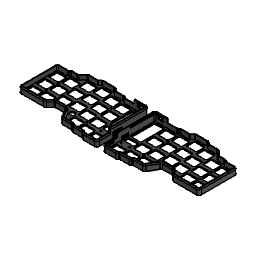
mriya-bumper-mjf-v1.09 (Autodesk Fusion 360 design; units mm, degrees)
Autodesk Fusion 360 part; units mm, degrees
(part 1 of 2)
sketch "mriya" plane through (0, 0, 0) normal (0, 0, 1) x (1, 0, 0)
  line L0 (-101.0213, 15.6719) -> (-94.7787, 21.9145) construction
  line L1 (-26.4858, 1.079) -> (-27.6142, 2.2074) construction
  line L2 (-138.1, 14.7932) -> (-103.1426, 14.7932) construction
  line L3 (-44.0716, 2.7932) -> (-29.0284, 2.7932) construction
  line L4 (-8.6, 0.4932) -> (-25.0716, 0.4932) construction
  line L5 (-64.4741, 6.1094) -> (-72.7517, 20.7608) construction
  line L6 (-45.4858, 3.379) -> (-46.6142, 4.5074) construction
  line L7 (-122.6142, 71.579) -> (-121.4858, 72.7074) construction
  line L8 (-101.0716, 81.2932) -> (-87.2284, 81.2932) construction
  line L9 (-138.1, 70.9932) -> (-124.0284, 70.9932) construction
  line L10 (-92.6574, 22.7932) -> (-76.2344, 22.7932) construction
  line L11 (-48.0284, 5.0932) -> (-62.7328, 5.0932) construction
  line L12 (-82.0716, 84.7932) -> (-64.7284, 84.7932) construction
  line L13 (-58.5716, 80.2932) -> (-45.7284, 80.2932) construction
  line L14 (-24.1, 19.4932) -> (-7.1, 19.4932) construction
  line L15 (-25.6, 20.9932) -> (-25.6, 77.9932) construction
  line L16 (-83.4858, 84.2074) -> (-85.8142, 81.879) construction
  line L17 (-63.3142, 84.2074) -> (-59.9858, 80.879) construction
  line L18 (-139.6, 69.4932) -> (-139.6, 16.2932) construction
  line L19 (-43.1858, 78.579) -> (-44.3142, 79.7074) construction
  line L20 (-99.4, 40.3932) -> (-99.4, 27.9932) construction
  line L21 (-98.6, 41.1932) -> (-86.2, 41.1932) construction
  line L22 (-98.6, 27.1932) -> (-86.2, 27.1932) construction
  line L23 (-85.4, 40.3932) -> (-85.4, 27.9932) construction
  line L24 (-42.4, 56.0932) -> (-42.4, 43.6932) construction
  line L25 (-41.6, 56.8932) -> (-29.2, 56.8932) construction
  line L26 (-41.6, 42.8932) -> (-29.2, 42.8932) construction
  line L27 (-28.4, 56.0932) -> (-28.4, 43.6932) construction
  line L28 (-61.4, 58.3932) -> (-61.4, 45.9932) construction
  line L29 (-60.6, 59.1932) -> (-48.2, 59.1932) construction
  line L30 (-60.6, 45.1932) -> (-48.2, 45.1932) construction
  line L31 (-47.4, 58.3932) -> (-47.4, 45.9932) construction
  line L32 (-137.4, 68.0932) -> (-137.4, 55.6932) construction
  line L33 (-136.6, 68.8932) -> (-124.2, 68.8932) construction
  line L34 (-136.6, 54.8932) -> (-124.2, 54.8932) construction
  line L35 (-123.4, 68.0932) -> (-123.4, 55.6932) construction
  line L36 (-61.4, 39.3932) -> (-61.4, 26.9932) construction
  line L37 (-60.6, 40.1932) -> (-48.2, 40.1932) construction
  line L38 (-60.6, 26.1932) -> (-48.2, 26.1932) construction
  line L39 (-47.4, 39.3932) -> (-47.4, 26.9932) construction
  line L40 (-42.4, 18.0932) -> (-42.4, 5.6932) construction
  line L41 (-41.6, 18.8932) -> (-29.2, 18.8932) construction
  line L42 (-41.6, 4.8932) -> (-29.2, 4.8932) construction
  line L43 (-28.4, 18.0932) -> (-28.4, 5.6932) construction
  line L44 (-23.4, 15.7932) -> (-23.4, 3.3932) construction
  line L45 (-22.6, 16.5932) -> (-10.2, 16.5932) construction
  line L46 (-22.6, 2.5932) -> (-10.2, 2.5932) construction
  line L47 (-9.4, 15.7932) -> (-9.4, 3.3932) construction
  line L48 (-137.4, 49.0932) -> (-137.4, 36.6932) construction
  line L49 (-136.6, 49.8932) -> (-124.2, 49.8932) construction
  line L50 (-136.6, 35.8932) -> (-124.2, 35.8932) construction
  line L51 (-123.4, 49.0932) -> (-123.4, 36.6932) construction
  line L52 (-118.4, 51.3932) -> (-118.4, 38.9932) construction
  line L53 (-117.6, 52.1932) -> (-105.2, 52.1932) construction
  line L54 (-117.6, 38.1932) -> (-105.2, 38.1932) construction
  line L55 (-104.4, 51.3932) -> (-104.4, 38.9932) construction
  line L56 (-137.4, 30.0932) -> (-137.4, 17.6932) construction
  line L57 (-136.6, 30.8932) -> (-124.2, 30.8932) construction
  line L58 (-136.6, 16.8932) -> (-124.2, 16.8932) construction
  line L59 (-123.4, 30.0932) -> (-123.4, 17.6932) construction
  line L60 (-61.4, 20.3932) -> (-61.4, 7.9932) construction
  line L61 (-60.6, 21.1932) -> (-48.2, 21.1932) construction
  line L62 (-60.6, 7.1932) -> (-48.2, 7.1932) construction
  line L63 (-47.4, 20.3932) -> (-47.4, 7.9932) construction
  line L64 (-80.4, 43.8932) -> (-80.4, 31.4932) construction
  line L65 (-79.6, 44.6932) -> (-67.2, 44.6932) construction
  line L66 (-79.6, 30.6932) -> (-67.2, 30.6932) construction
  line L67 (-66.4, 43.8932) -> (-66.4, 31.4932) construction
  line L68 (-80.4, 81.8932) -> (-80.4, 69.4932) construction
  line L69 (-79.6, 82.6932) -> (-67.2, 82.6932) construction
  line L70 (-79.6, 68.6932) -> (-67.2, 68.6932) construction
  line L71 (-66.4, 81.8932) -> (-66.4, 69.4932) construction
  line L72 (-42.4, 37.0932) -> (-42.4, 24.6932) construction
  line L73 (-41.6, 37.8932) -> (-29.2, 37.8932) construction
  line L74 (-41.6, 23.8932) -> (-29.2, 23.8932) construction
  line L75 (-28.4, 37.0932) -> (-28.4, 24.6932) construction
  line L76 (-118.4, 32.3932) -> (-118.4, 19.9932) construction
  line L77 (-117.6, 33.1932) -> (-105.2, 33.1932) construction
  line L78 (-117.6, 19.1932) -> (-105.2, 19.1932) construction
  line L79 (-104.4, 32.3932) -> (-104.4, 19.9932) construction
  line L80 (-61.4, 77.3932) -> (-61.4, 64.9932) construction
  line L81 (-60.6, 78.1932) -> (-48.2, 78.1932) construction
  line L82 (-60.6, 64.1932) -> (-48.2, 64.1932) construction
  line L83 (-47.4, 77.3932) -> (-47.4, 64.9932) construction
  line L84 (-42.4, 75.0932) -> (-42.4, 62.6932) construction
  line L85 (-41.6, 75.8932) -> (-29.2, 75.8932) construction
  line L86 (-41.6, 61.8932) -> (-29.2, 61.8932) construction
  line L87 (-28.4, 75.0932) -> (-28.4, 62.6932) construction
  line L88 (-118.4, 70.3932) -> (-118.4, 57.9932) construction
  line L89 (-117.6, 71.1932) -> (-105.2, 71.1932) construction
  line L90 (-117.6, 57.1932) -> (-105.2, 57.1932) construction
  line L91 (-104.4, 70.3932) -> (-104.4, 57.9932) construction
  line L92 (-99.4, 59.3932) -> (-99.4, 46.9932) construction
  line L93 (-98.6, 60.1932) -> (-86.2, 60.1932) construction
  line L94 (-98.6, 46.1932) -> (-86.2, 46.1932) construction
  line L95 (-85.4, 59.3932) -> (-85.4, 46.9932) construction
  line L96 (-80.4, 62.8932) -> (-80.4, 50.4932) construction
  line L97 (-79.6, 63.6932) -> (-67.2, 63.6932) construction
  line L98 (-79.6, 49.6932) -> (-67.2, 49.6932) construction
  line L99 (-66.4, 62.8932) -> (-66.4, 50.4932) construction
  line L100 (-99.4, 78.3932) -> (-99.4, 65.9932) construction
  line L101 (-98.6, 79.1932) -> (-86.2, 79.1932) construction
  line L102 (-98.6, 65.1932) -> (-86.2, 65.1932) construction
  line L103 (-85.4, 78.3932) -> (-85.4, 65.9932) construction
  circle A0 centre (-120.9, 53.5432) radius 1.65
  circle A1 centre (-120.9, 34.5432) radius 1.65
  circle A2 centre (-68.5, 23.5932) radius 4
  circle A3 centre (-44.9, 22.5432) radius 1.65
  circle A4 centre (-44.9, 60.5432) radius 1.65
  arc A5 (-43.1858, 78.579) -> (-41.7716, 77.9932) centre (-41.7716, 79.9932) ccw construction
  arc A6 (-44.3142, 79.7074) -> (-45.7284, 80.2932) centre (-45.7285, 78.2931) ccw construction
  arc A7 (-59.9858, 80.879) -> (-58.5716, 80.2932) centre (-58.5716, 82.2931) ccw construction
  arc A8 (-63.3142, 84.2074) -> (-64.7284, 84.7932) centre (-64.7285, 82.7931) ccw construction
  arc A9 (-82.0716, 84.7932) -> (-83.4858, 84.2074) centre (-82.0716, 82.7933) ccw construction
  arc A10 (-87.2284, 81.2932) -> (-85.8142, 81.879) centre (-87.2284, 83.2932) ccw construction
  arc A11 (-101.0716, 81.2932) -> (-102.4858, 80.7074) centre (-101.0716, 79.2933) ccw construction
  arc A12 (-120.0716, 73.2932) -> (-121.4858, 72.7074) centre (-120.0716, 71.2933) ccw construction
  arc A13 (-124.0284, 70.9932) -> (-122.6142, 71.579) centre (-124.0284, 72.9932) ccw construction
  arc A14 (-138.1, 70.9932) -> (-139.6, 69.4932) centre (-138.1, 69.4932) ccw construction
  arc A15 (-139.6, 16.2932) -> (-138.1, 14.7932) centre (-138.1, 16.2932) ccw construction
  arc A16 (-103.1426, 14.7932) -> (-101.0213, 15.6719) centre (-103.1426, 17.7931) ccw construction
  arc A17 (-92.6574, 22.7932) -> (-94.7787, 21.9145) centre (-92.6573, 19.7931) ccw construction
  arc A18 (-72.7517, 20.7608) -> (-76.2344, 22.7932) centre (-76.2344, 18.793) ccw construction
  arc A19 (-64.4741, 6.1094) -> (-62.7328, 5.0932) centre (-62.7328, 7.0932) ccw construction
  arc A20 (-46.6142, 4.5074) -> (-48.0284, 5.0932) centre (-48.0284, 3.0933) ccw construction
  arc A21 (-45.4858, 3.379) -> (-44.0716, 2.7932) centre (-44.0715, 4.7933) ccw construction
  arc A22 (-27.6142, 2.2074) -> (-29.0284, 2.7932) centre (-29.0284, 0.7933) ccw construction
  arc A23 (-26.4858, 1.079) -> (-25.0716, 0.4932) centre (-25.0715, 2.4933) ccw construction
  arc A24 (-8.6, 0.4932) -> (-7.1, 1.9932) centre (-8.6, 1.9932) ccw construction
  arc A25 (-25.6, 20.9932) -> (-24.1, 19.4932) centre (-24.1, 20.9932) ccw construction
  line L104 (-7.1, 1.9932) -> (-7.1, 76.4932) construction
  line L105 (-41.7716, 77.9932) -> (-8.6, 77.9932) construction
  arc A26 (-7.1, 76.4932) -> (-8.6, 77.9932) centre (-8.6, 76.4932) ccw construction
  arc A27 (-136.6, 68.8932) -> (-137.4, 68.0932) centre (-136.6, 68.0932) ccw construction
  arc A28 (-123.4, 68.0932) -> (-124.2, 68.8932) centre (-124.2, 68.0932) ccw construction
  arc A29 (-124.2, 54.8932) -> (-123.4, 55.6932) centre (-124.2, 55.6932) ccw construction
  arc A30 (-137.4, 55.6932) -> (-136.6, 54.8932) centre (-136.6, 55.6932) ccw construction
  arc A31 (-136.6, 49.8932) -> (-137.4, 49.0932) centre (-136.6, 49.0932) ccw construction
  arc A32 (-123.4, 49.0932) -> (-124.2, 49.8932) centre (-124.2, 49.0932) ccw construction
  arc A33 (-124.2, 35.8932) -> (-123.4, 36.6932) centre (-124.2, 36.6932) ccw construction
  arc A34 (-137.4, 36.6932) -> (-136.6, 35.8932) centre (-136.6, 36.6932) ccw construction
  arc A35 (-136.6, 30.8932) -> (-137.4, 30.0932) centre (-136.6, 30.0932) ccw construction
  arc A36 (-123.4, 30.0932) -> (-124.2, 30.8932) centre (-124.2, 30.0932) ccw construction
  arc A37 (-124.2, 16.8932) -> (-123.4, 17.6932) centre (-124.2, 17.6932) ccw construction
  arc A38 (-137.4, 17.6932) -> (-136.6, 16.8932) centre (-136.6, 17.6932) ccw construction
  arc A39 (-118.4, 19.9932) -> (-117.6, 19.1932) centre (-117.6, 19.9932) ccw construction
  arc A40 (-105.2, 19.1932) -> (-104.4, 19.9932) centre (-105.2, 19.9932) ccw construction
  arc A41 (-104.4, 32.3932) -> (-105.2, 33.1932) centre (-105.2, 32.3932) ccw construction
  arc A42 (-117.6, 33.1932) -> (-118.4, 32.3932) centre (-117.6, 32.3932) ccw construction
  arc A43 (-105.2, 38.1932) -> (-104.4, 38.9932) centre (-105.2, 38.9932) ccw construction
  arc A44 (-118.4, 38.9932) -> (-117.6, 38.1932) centre (-117.6, 38.9932) ccw construction
  arc A45 (-117.6, 52.1932) -> (-118.4, 51.3932) centre (-117.6, 51.3932) ccw construction
  arc A46 (-104.4, 51.3932) -> (-105.2, 52.1932) centre (-105.2, 51.3932) ccw construction
  arc A47 (-118.4, 57.9932) -> (-117.6, 57.1932) centre (-117.6, 57.9932) ccw construction
  arc A48 (-105.2, 57.1932) -> (-104.4, 57.9932) centre (-105.2, 57.9932) ccw construction
  arc A49 (-104.4, 70.3932) -> (-105.2, 71.1932) centre (-105.2, 70.3932) ccw construction
  arc A50 (-117.6, 71.1932) -> (-118.4, 70.3932) centre (-117.6, 70.3932) ccw construction
  arc A51 (-98.6, 79.1932) -> (-99.4, 78.3932) centre (-98.6, 78.3932) ccw construction
  arc A52 (-85.4, 78.3932) -> (-86.2, 79.1932) centre (-86.2, 78.3932) ccw construction
  arc A53 (-86.2, 65.1932) -> (-85.4, 65.9932) centre (-86.2, 65.9932) ccw construction
  arc A54 (-99.4, 65.9932) -> (-98.6, 65.1932) centre (-98.6, 65.9932) ccw construction
  arc A55 (-98.6, 60.1932) -> (-99.4, 59.3932) centre (-98.6, 59.3932) ccw construction
  arc A56 (-85.4, 59.3932) -> (-86.2, 60.1932) centre (-86.2, 59.3932) ccw construction
  arc A57 (-86.2, 46.1932) -> (-85.4, 46.9932) centre (-86.2, 46.9932) ccw construction
  arc A58 (-99.4, 46.9932) -> (-98.6, 46.1932) centre (-98.6, 46.9932) ccw construction
  arc A59 (-98.6, 41.1932) -> (-99.4, 40.3932) centre (-98.6, 40.3932) ccw construction
  arc A60 (-99.4, 27.9932) -> (-98.6, 27.1932) centre (-98.6, 27.9932) ccw construction
  arc A61 (-86.2, 27.1932) -> (-85.4, 27.9932) centre (-86.2, 27.9932) ccw construction
  arc A62 (-85.4, 40.3932) -> (-86.2, 41.1932) centre (-86.2, 40.3932) ccw construction
  arc A63 (-80.4, 31.4932) -> (-79.6, 30.6932) centre (-79.6, 31.4932) ccw construction
  arc A64 (-79.6, 44.6932) -> (-80.4, 43.8932) centre (-79.6, 43.8932) ccw construction
  arc A65 (-66.4, 43.8932) -> (-67.2, 44.6932) centre (-67.2, 43.8932) ccw construction
  arc A66 (-67.2, 30.6932) -> (-66.4, 31.4932) centre (-67.2, 31.4932) ccw construction
  arc A67 (-67.2, 49.6932) -> (-66.4, 50.4932) centre (-67.2, 50.4932) ccw construction
  arc A68 (-80.4, 50.4932) -> (-79.6, 49.6932) centre (-79.6, 50.4932) ccw construction
  arc A69 (-79.6, 63.6932) -> (-80.4, 62.8932) centre (-79.6, 62.8932) ccw construction
  arc A70 (-66.4, 62.8932) -> (-67.2, 63.6932) centre (-67.2, 62.8932) ccw construction
  arc A71 (-67.2, 68.6932) -> (-66.4, 69.4932) centre (-67.2, 69.4932) ccw construction
  arc A72 (-80.4, 69.4932) -> (-79.6, 68.6932) centre (-79.6, 69.4932) ccw construction
  arc A73 (-79.6, 82.6932) -> (-80.4, 81.8932) centre (-79.6, 81.8932) ccw construction
  arc A74 (-66.4, 81.8932) -> (-67.2, 82.6932) centre (-67.2, 81.8932) ccw construction
  arc A75 (-60.6, 78.1932) -> (-61.4, 77.3932) centre (-60.6, 77.3932) ccw construction
  arc A76 (-61.4, 64.9932) -> (-60.6, 64.1932) centre (-60.6, 64.9932) ccw construction
  arc A77 (-48.2, 64.1932) -> (-47.4, 64.9932) centre (-48.2, 64.9932) ccw construction
  arc A78 (-47.4, 77.3932) -> (-48.2, 78.1932) centre (-48.2, 77.3932) ccw construction
  arc A79 (-47.4, 58.3932) -> (-48.2, 59.1932) centre (-48.2, 58.3932) ccw construction
  arc A80 (-60.6, 59.1932) -> (-61.4, 58.3932) centre (-60.6, 58.3932) ccw construction
  arc A81 (-61.4, 45.9932) -> (-60.6, 45.1932) centre (-60.6, 45.9932) ccw construction
  arc A82 (-48.2, 45.1932) -> (-47.4, 45.9932) centre (-48.2, 45.9932) ccw construction
  arc A83 (-47.4, 39.3932) -> (-48.2, 40.1932) centre (-48.2, 39.3932) ccw construction
  arc A84 (-60.6, 40.1932) -> (-61.4, 39.3932) centre (-60.6, 39.3932) ccw construction
  arc A85 (-61.4, 26.9932) -> (-60.6, 26.1932) centre (-60.6, 26.9932) ccw construction
  arc A86 (-48.2, 26.1932) -> (-47.4, 26.9932) centre (-48.2, 26.9932) ccw construction
  arc A87 (-47.4, 20.3932) -> (-48.2, 21.1932) centre (-48.2, 20.3932) ccw construction
  arc A88 (-60.6, 21.1932) -> (-61.4, 20.3932) centre (-60.6, 20.3932) ccw construction
  arc A89 (-61.4, 7.9932) -> (-60.6, 7.1932) centre (-60.6, 7.9932) ccw construction
  arc A90 (-48.2, 7.1932) -> (-47.4, 7.9932) centre (-48.2, 7.9932) ccw construction
  arc A91 (-42.4, 5.6932) -> (-41.6, 4.8932) centre (-41.6, 5.6932) ccw construction
  arc A92 (-29.2, 4.8932) -> (-28.4, 5.6932) centre (-29.2, 5.6932) ccw construction
  arc A93 (-28.4, 18.0932) -> (-29.2, 18.8932) centre (-29.2, 18.0932) ccw construction
  arc A94 (-41.6, 18.8932) -> (-42.4, 18.0932) centre (-41.6, 18.0932) ccw construction
  arc A95 (-23.4, 3.3932) -> (-22.6, 2.5932) centre (-22.6, 3.3932) ccw construction
  arc A96 (-10.2, 2.5932) -> (-9.4, 3.3932) centre (-10.2, 3.3932) ccw construction
  arc A97 (-9.4, 15.7932) -> (-10.2, 16.5932) centre (-10.2, 15.7932) ccw construction
  arc A98 (-22.6, 16.5932) -> (-23.4, 15.7932) centre (-22.6, 15.7932) ccw construction
  arc A99 (-29.2, 23.8932) -> (-28.4, 24.6932) centre (-29.2, 24.6932) ccw construction
  arc A100 (-42.4, 24.6932) -> (-41.6, 23.8932) centre (-41.6, 24.6932) ccw construction
  arc A101 (-41.6, 37.8932) -> (-42.4, 37.0932) centre (-41.6, 37.0932) ccw construction
  arc A102 (-28.4, 37.0932) -> (-29.2, 37.8932) centre (-29.2, 37.0932) ccw construction
  arc A103 (-29.2, 42.8932) -> (-28.4, 43.6932) centre (-29.2, 43.6932) ccw construction
  arc A104 (-42.4, 43.6932) -> (-41.6, 42.8932) centre (-41.6, 43.6932) ccw construction
  arc A105 (-41.6, 56.8932) -> (-42.4, 56.0932) centre (-41.6, 56.0932) ccw construction
  arc A106 (-28.4, 56.0932) -> (-29.2, 56.8932) centre (-29.2, 56.0932) ccw construction
  arc A107 (-29.2, 61.8932) -> (-28.4, 62.6932) centre (-29.2, 62.6932) ccw construction
  arc A108 (-42.4, 62.6932) -> (-41.6, 61.8932) centre (-41.6, 62.6932) ccw construction
  arc A109 (-41.6, 75.8932) -> (-42.4, 75.0932) centre (-41.6, 75.0932) ccw construction
  arc A110 (-28.4, 75.0932) -> (-29.2, 75.8932) centre (-29.2, 75.0932) ccw construction
  circle A111 centre (-22.6, 22.4932) radius 1.1
  circle A112 centre (-10.1, 22.4932) radius 1.1
  line L106 (-7, 19.2932) -> (-4.5, 19.2932)
  line L107 (-25.8, 78.0932) -> (-25.8, 80.5932)
  line L108 (-20.3, 77.2932) -> (-8.6, 77.2932)
  line L109 (-7.8, 39.7932) -> (-7.8, 76.4932)
  line L110 (-7.8, 12.7932) -> (-7.8, 6.3932)
  line L111 (-102.4858, 80.7074) -> (-109.0213, 74.1719) construction
  line L112 (-120.0716, 73.2932) -> (-111.1426, 73.2932) construction
  arc A113 (-111.1426, 73.2932) -> (-109.0213, 74.1719) centre (-111.1426, 76.2932) ccw construction
  arc A114 (-64.7284, 82.7932) -> (-64.7285, 82.7932) centre (-64.7285, 82.7931) ccw
  arc A115 (-45.7284, 78.2932) -> (-45.7285, 78.2932) centre (-45.7285, 78.2931) ccw
  arc A116 (-25.0716, 2.4932) -> (-25.0715, 2.4932) centre (-25.0715, 2.4933) ccw
  arc A117 (-44.0716, 4.7932) -> (-44.0715, 4.7932) centre (-44.0715, 4.7933) ccw
  line L113 (-138.9, 56.8932) -> (-138.9, 66.8932)
  line L114 (-136.9, 68.8932) -> (-123.9, 68.8932)
  arc A118 (-121.9, 66.8932) -> (-123.9, 68.8932) centre (-123.9, 66.8932) ccw
  arc A119 (-138.9, 56.8932) -> (-136.9, 54.8932) centre (-136.9, 56.8932) ccw
  arc A120 (-136.9, 68.8932) -> (-138.9, 66.8932) centre (-136.9, 66.8932) ccw
  arc A121 (-138.9, 37.8932) -> (-136.9, 35.8932) centre (-136.9, 37.8932) ccw
  line L115 (-138.9, 37.8932) -> (-138.9, 47.8932)
  arc A122 (-136.9, 49.8932) -> (-138.9, 47.8932) centre (-136.9, 47.8932) ccw
  line L116 (-136.9, 49.8932) -> (-123.9, 49.8932)
  arc A123 (-121.9, 47.8932) -> (-123.9, 49.8932) centre (-123.9, 47.8932) ccw
  arc A124 (-123.9, 16.8932) -> (-121.9, 18.8932) centre (-123.9, 18.8932) ccw
  line L117 (-123.9, 16.8932) -> (-136.9, 16.8932)
  arc A125 (-138.9, 18.8932) -> (-136.9, 16.8932) centre (-136.9, 18.8932) ccw
  line L118 (-138.9, 18.8932) -> (-138.9, 28.8932)
  arc A126 (-136.9, 30.8932) -> (-138.9, 28.8932) centre (-136.9, 28.8932) ccw
  line L119 (-136.9, 30.8932) -> (-123.9, 30.8932)
  arc A127 (-121.9, 28.8932) -> (-123.9, 30.8932) centre (-123.9, 28.8932) ccw
  line L120 (-121.9, 28.8932) -> (-121.9, 18.8932)
  arc A128 (-104.9, 57.1932) -> (-102.9, 59.1932) centre (-104.9, 59.1932) ccw
  line L121 (-104.9, 57.1932) -> (-117.9, 57.1932)
  arc A129 (-119.9, 59.1932) -> (-117.9, 57.1932) centre (-117.9, 59.1932) ccw
  line L122 (-119.9, 59.1932) -> (-119.9, 69.1932)
  arc A130 (-117.9, 71.1932) -> (-119.9, 69.1932) centre (-117.9, 69.1932) ccw
  line L123 (-117.9, 71.1932) -> (-104.9, 71.1932)
  arc A131 (-102.9, 69.1932) -> (-104.9, 71.1932) centre (-104.9, 69.1932) ccw
  line L124 (-102.9, 69.1932) -> (-102.9, 59.1932)
  arc A132 (-104.9, 38.1932) -> (-102.9, 40.1932) centre (-104.9, 40.1932) ccw
  line L125 (-104.9, 38.1932) -> (-117.9, 38.1932)
  arc A133 (-119.9, 40.1932) -> (-117.9, 38.1932) centre (-117.9, 40.1932) ccw
  arc A134 (-102.9, 50.1932) -> (-104.9, 52.1932) centre (-104.9, 50.1932) ccw
  line L126 (-102.9, 50.1932) -> (-102.9, 40.1932)
  arc A135 (-104.9, 19.1932) -> (-102.9, 21.1932) centre (-104.9, 21.1932) ccw
  line L127 (-104.9, 19.1932) -> (-117.9, 19.1932)
  arc A136 (-119.9, 21.1932) -> (-117.9, 19.1932) centre (-117.9, 21.1932) ccw
  arc A137 (-102.9, 31.1932) -> (-104.9, 33.1932) centre (-104.9, 31.1932) ccw
  line L128 (-102.9, 31.1932) -> (-102.9, 21.1932)
  arc A138 (-85.9, 65.1932) -> (-83.9, 67.1932) centre (-85.9, 67.1932) ccw
  line L129 (-85.9, 65.1932) -> (-98.9, 65.1932)
  arc A139 (-100.9, 67.1932) -> (-98.9, 65.1932) centre (-98.9, 67.1932) ccw
  line L130 (-100.9, 67.1932) -> (-100.9, 77.1932)
  arc A140 (-98.9, 79.1932) -> (-100.9, 77.1932) centre (-98.9, 77.1932) ccw
  line L131 (-98.9, 79.1932) -> (-85.9, 79.1932)
  arc A141 (-83.9, 77.1932) -> (-85.9, 79.1932) centre (-85.9, 77.1932) ccw
  line L132 (-83.9, 77.1932) -> (-83.9, 67.1932)
  arc A142 (-85.9, 46.1932) -> (-83.9, 48.1932) centre (-85.9, 48.1932) ccw
  line L133 (-85.9, 46.1932) -> (-98.9, 46.1932)
  arc A143 (-100.9, 48.1932) -> (-98.9, 46.1932) centre (-98.9, 48.1932) ccw
  line L134 (-100.9, 48.1932) -> (-100.9, 58.1932)
  arc A144 (-98.9, 60.1932) -> (-100.9, 58.1932) centre (-98.9, 58.1932) ccw
  line L135 (-98.9, 60.1932) -> (-85.9, 60.1932)
  arc A145 (-83.9, 58.1932) -> (-85.9, 60.1932) centre (-85.9, 58.1932) ccw
  line L136 (-83.9, 58.1932) -> (-83.9, 48.1932)
  arc A146 (-85.9, 27.1932) -> (-83.9, 29.1932) centre (-85.9, 29.1932) ccw
  line L137 (-85.9, 27.1932) -> (-98.9, 27.1932)
  arc A147 (-100.9, 29.1932) -> (-98.9, 27.1932) centre (-98.9, 29.1932) ccw
  line L138 (-100.9, 29.1932) -> (-100.9, 39.1932)
  arc A148 (-98.9, 41.1932) -> (-100.9, 39.1932) centre (-98.9, 39.1932) ccw
  line L139 (-98.9, 41.1932) -> (-85.9, 41.1932)
  arc A149 (-83.9, 39.1932) -> (-85.9, 41.1932) centre (-85.9, 39.1932) ccw
  line L140 (-83.9, 39.1932) -> (-83.9, 29.1932)
  arc A150 (-66.9, 30.6932) -> (-64.9, 32.6932) centre (-66.9, 32.6932) ccw
  line L141 (-66.9, 30.6932) -> (-79.9, 30.6932)
  arc A151 (-81.9, 32.6932) -> (-79.9, 30.6932) centre (-79.9, 32.6932) ccw
  line L142 (-81.9, 32.6932) -> (-81.9, 42.6932)
  arc A152 (-79.9, 44.6932) -> (-81.9, 42.6932) centre (-79.9, 42.6932) ccw
  line L143 (-79.9, 44.6932) -> (-66.9, 44.6932)
  arc A153 (-64.9, 42.6932) -> (-66.9, 44.6932) centre (-66.9, 42.6932) ccw
  line L144 (-64.9, 42.6932) -> (-64.9, 32.6932)
  arc A154 (-66.9, 49.6932) -> (-64.9, 51.6932) centre (-66.9, 51.6932) ccw
  line L145 (-66.9, 49.6932) -> (-79.9, 49.6932)
  arc A155 (-81.9, 51.6932) -> (-79.9, 49.6932) centre (-79.9, 51.6932) ccw
  line L146 (-81.9, 51.6932) -> (-81.9, 61.6932)
  arc A156 (-79.9, 63.6932) -> (-81.9, 61.6932) centre (-79.9, 61.6932) ccw
  line L147 (-79.9, 63.6932) -> (-66.9, 63.6932)
  arc A157 (-64.9, 61.6932) -> (-66.9, 63.6932) centre (-66.9, 61.6932) ccw
  line L148 (-64.9, 61.6932) -> (-64.9, 51.6932)
  arc A158 (-66.9, 68.6932) -> (-64.9, 70.6932) centre (-66.9, 70.6932) ccw
  line L149 (-66.9, 68.6932) -> (-79.9, 68.6932)
  arc A159 (-81.9, 70.6932) -> (-79.9, 68.6932) centre (-79.9, 70.6932) ccw
  line L150 (-81.9, 70.6932) -> (-81.9, 80.6932)
  arc A160 (-79.9, 82.6932) -> (-81.9, 80.6932) centre (-79.9, 80.6932) ccw
  line L151 (-79.9, 82.6932) -> (-66.9, 82.6932)
  arc A161 (-64.9, 80.6932) -> (-66.9, 82.6932) centre (-66.9, 80.6932) ccw
  line L152 (-64.9, 80.6932) -> (-64.9, 70.6932)
  arc A162 (-47.9, 26.1932) -> (-45.9, 28.1932) centre (-47.9, 28.1932) ccw
  line L153 (-47.9, 26.1932) -> (-60.9, 26.1932)
  arc A163 (-62.9, 28.1932) -> (-60.9, 26.1932) centre (-60.9, 28.1932) ccw
  line L154 (-62.9, 28.1932) -> (-62.9, 38.1932)
  arc A164 (-60.9, 40.1932) -> (-62.9, 38.1932) centre (-60.9, 38.1932) ccw
  line L155 (-60.9, 40.1932) -> (-47.9, 40.1932)
  arc A165 (-45.9, 38.1932) -> (-47.9, 40.1932) centre (-47.9, 38.1932) ccw
  line L156 (-45.9, 38.1932) -> (-45.9, 28.1932)
  arc A166 (-47.9, 45.1932) -> (-45.9, 47.1932) centre (-47.9, 47.1932) ccw
  line L157 (-47.9, 45.1932) -> (-60.9, 45.1932)
  arc A167 (-62.9, 47.1932) -> (-60.9, 45.1932) centre (-60.9, 47.1932) ccw
  line L158 (-62.9, 47.1932) -> (-62.9, 57.1932)
  arc A168 (-60.9, 59.1932) -> (-62.9, 57.1932) centre (-60.9, 57.1932) ccw
  arc A169 (-47.9, 64.1932) -> (-45.9, 66.1932) centre (-47.9, 66.1932) ccw
  line L159 (-47.9, 64.1932) -> (-60.9, 64.1932)
  arc A170 (-62.9, 66.1932) -> (-60.9, 64.1932) centre (-60.9, 66.1932) ccw
  line L160 (-62.9, 66.1932) -> (-62.9, 76.1932)
  arc A171 (-60.9, 78.1932) -> (-62.9, 76.1932) centre (-60.9, 76.1932) ccw
  line L161 (-60.9, 78.1932) -> (-47.9, 78.1932)
  arc A172 (-45.9, 76.1932) -> (-47.9, 78.1932) centre (-47.9, 76.1932) ccw
  line L162 (-45.9, 76.1932) -> (-45.9, 66.1932)
  arc A173 (-47.9, 7.1932) -> (-45.9, 9.1932) centre (-47.9, 9.1932) ccw
  line L163 (-47.9, 7.1932) -> (-60.9, 7.1932)
  arc A174 (-62.9, 9.1932) -> (-60.9, 7.1932) centre (-60.9, 9.1932) ccw
  line L164 (-62.9, 9.1932) -> (-62.9, 19.1932)
  arc A175 (-60.9, 21.1932) -> (-62.9, 19.1932) centre (-60.9, 19.1932) ccw
  arc A176 (-28.9, 4.8932) -> (-26.9, 6.8932) centre (-28.9, 6.8932) ccw
  line L165 (-28.9, 4.8932) -> (-41.9, 4.8932)
  arc A177 (-43.9, 6.8932) -> (-41.9, 4.8932) centre (-41.9, 6.8932) ccw
  line L166 (-43.9, 6.8932) -> (-43.9, 16.8932)
  arc A178 (-41.9, 18.8932) -> (-43.9, 16.8932) centre (-41.9, 16.8932) ccw
  line L167 (-41.9, 18.8932) -> (-28.9, 18.8932)
  arc A179 (-26.9, 16.8932) -> (-28.9, 18.8932) centre (-28.9, 16.8932) ccw
  line L168 (-26.9, 16.8932) -> (-26.9, 6.8932)
  arc A180 (-28.9, 23.8932) -> (-26.9, 25.8932) centre (-28.9, 25.8932) ccw
  arc A181 (-41.9, 37.8932) -> (-43.9, 35.8932) centre (-41.9, 35.8932) ccw
  line L169 (-41.9, 37.8932) -> (-28.9, 37.8932)
  arc A182 (-26.9, 35.8932) -> (-28.9, 37.8932) centre (-28.9, 35.8932) ccw
  line L170 (-26.9, 35.8932) -> (-26.9, 25.8932)
  arc A183 (-28.9, 42.8932) -> (-26.9, 44.8932) centre (-28.9, 44.8932) ccw
  line L171 (-28.9, 42.8932) -> (-41.9, 42.8932)
  arc A184 (-43.9, 44.8932) -> (-41.9, 42.8932) centre (-41.9, 44.8932) ccw
  line L172 (-43.9, 44.8932) -> (-43.9, 54.8932)
  arc A185 (-41.9, 56.8932) -> (-43.9, 54.8932) centre (-41.9, 54.8932) ccw
  line L173 (-41.9, 56.8932) -> (-28.9, 56.8932)
  arc A186 (-26.9, 54.8932) -> (-28.9, 56.8932) centre (-28.9, 54.8932) ccw
  line L174 (-26.9, 54.8932) -> (-26.9, 44.8932)
  arc A187 (-28.9, 61.8932) -> (-26.9, 63.8932) centre (-28.9, 63.8932) ccw
  line L175 (-43.9, 64.3145) -> (-43.9, 73.8932)
  arc A188 (-41.9, 75.8932) -> (-43.9, 73.8932) centre (-41.9, 73.8932) ccw
  line L176 (-41.9, 75.8932) -> (-28.9, 75.8932)
  arc A189 (-26.9, 73.8932) -> (-28.9, 75.8932) centre (-28.9, 73.8932) ccw
  line L177 (-26.9, 73.8932) -> (-26.9, 63.8932)
  arc A190 (-9.9, 2.5932) -> (-7.9, 4.5932) centre (-9.9, 4.5932) ccw
  line L178 (-9.9, 2.5932) -> (-22.9, 2.5932)
  arc A191 (-24.9, 4.5932) -> (-22.9, 2.5932) centre (-22.9, 4.5932) ccw
  line L179 (-24.9, 4.5932) -> (-24.9, 14.5932)
  arc A192 (-22.9, 16.5932) -> (-24.9, 14.5932) centre (-22.9, 14.5932) ccw
  line L180 (-22.9, 16.5932) -> (-9.9, 16.5932)
  arc A193 (-7.9, 14.5932) -> (-9.9, 16.5932) centre (-9.9, 14.5932) ccw
  line L181 (-7.9, 14.5932) -> (-7.9, 4.5932)
  arc A194 (-9.9, 26.8932) -> (-7.9, 28.8932) centre (-9.9, 28.8932) ccw
  line L182 (-9.9, 26.8932) -> (-22.9, 26.8932)
  arc A195 (-24.9, 28.8932) -> (-22.9, 26.8932) centre (-22.9, 28.8932) ccw
  arc A196 (-22.9, 75.8932) -> (-24.9, 73.8932) centre (-22.9, 73.8932) ccw
  line L183 (-22.9, 75.8932) -> (-9.9, 75.8932)
  arc A197 (-7.9, 73.8932) -> (-9.9, 75.8932) centre (-9.9, 73.8932) ccw
  line L184 (-43.9, 26.3145) -> (-43.9, 35.8932)
  line L185 (-28.9, 23.8932) -> (-41.4787, 23.8932)
  line L186 (-43.4607, 25.2539) -> (-42.5393, 24.3325)
  line L187 (-60.9, 21.1932) -> (-48.3213, 21.1932)
  line L188 (-45.9, 18.7719) -> (-45.9, 9.1932)
  line L189 (-47.2607, 20.7539) -> (-46.3393, 19.8325)
  line L190 (-60.9, 59.1932) -> (-48.3213, 59.1932)
  line L191 (-45.9, 56.7719) -> (-45.9, 47.1932)
  line L192 (-28.9, 61.8932) -> (-41.4787, 61.8932)
  line L193 (-47.2607, 58.7539) -> (-46.3393, 57.8325)
  line L194 (-42.5393, 62.3325) -> (-43.4607, 63.2539)
  line L195 (-121.9, 66.8932) -> (-121.9, 57.3145)
  line L196 (-124.3213, 54.8932) -> (-136.9, 54.8932)
  line L197 (-117.4787, 52.1932) -> (-104.9, 52.1932)
  line L198 (-119.9, 40.1932) -> (-119.9, 49.7719)
  line L199 (-123.2607, 55.3325) -> (-122.3393, 56.2539)
  line L200 (-118.5393, 51.7539) -> (-119.4607, 50.8325)
  line L201 (-119.9, 21.1932) -> (-119.9, 30.7719)
  line L202 (-117.4787, 33.1932) -> (-104.9, 33.1932)
  line L203 (-121.9, 47.8932) -> (-121.9, 38.3145)
  line L204 (-124.3213, 35.8932) -> (-136.9, 35.8932)
  line L205 (-123.2607, 36.3325) -> (-122.3393, 37.2539)
  line L206 (-119.4607, 31.8325) -> (-118.5393, 32.7539)
  arc A198 (-43.9, 26.3145) -> (-43.4607, 25.2539) centre (-42.4, 26.3145) ccw
  arc A199 (-42.5393, 24.3325) -> (-41.4787, 23.8932) centre (-41.4787, 25.3932) ccw
  arc A200 (-47.2607, 20.7539) -> (-48.3213, 21.1932) centre (-48.3213, 19.6932) ccw
  arc A201 (-45.9, 18.7719) -> (-46.3393, 19.8325) centre (-47.4, 18.7719) ccw
  arc A202 (-47.2607, 58.7539) -> (-48.3213, 59.1932) centre (-48.3213, 57.6932) ccw
  arc A203 (-45.9, 56.7719) -> (-46.3393, 57.8325) centre (-47.4, 56.7719) ccw
  arc A204 (-42.5393, 62.3325) -> (-41.4787, 61.8932) centre (-41.4787, 63.3932) ccw
  arc A205 (-43.9, 64.3145) -> (-43.4607, 63.2539) centre (-42.4, 64.3145) ccw
  arc A206 (-122.3393, 56.2539) -> (-121.9, 57.3145) centre (-123.4, 57.3145) ccw
  arc A207 (-124.3213, 54.8932) -> (-123.2607, 55.3325) centre (-124.3213, 56.3932) ccw
  arc A208 (-117.4787, 52.1932) -> (-118.5393, 51.7539) centre (-117.4787, 50.6932) ccw
  arc A209 (-119.4607, 50.8325) -> (-119.9, 49.7719) centre (-118.4, 49.7719) ccw
  arc A210 (-122.3393, 37.2539) -> (-121.9, 38.3145) centre (-123.4, 38.3145) ccw
  arc A211 (-124.3213, 35.8932) -> (-123.2607, 36.3325) centre (-124.3213, 37.3932) ccw
  arc A212 (-119.4607, 31.8325) -> (-119.9, 30.7719) centre (-118.4, 30.7719) ccw
  arc A213 (-117.4787, 33.1932) -> (-118.5393, 32.7539) centre (-117.4787, 31.6932) ccw
  line L207 (-122.6849, 71.6497) -> (-121.5565, 72.7781)
  arc A214 (-120.0716, 73.3932) -> (-121.5565, 72.7781) centre (-120.0716, 71.2933) ccw
  line L208 (-120.0716, 73.3932) -> (-111.1426, 73.3932)
  arc A215 (-111.1426, 73.3932) -> (-109.092, 74.2426) centre (-111.1426, 76.2932) ccw
  line L209 (-102.5565, 80.7781) -> (-109.092, 74.2426)
  arc A216 (-101.0716, 81.3932) -> (-102.5565, 80.7781) centre (-101.0716, 79.2933) ccw
  line L210 (-101.0716, 81.3932) -> (-87.2284, 81.3932)
  arc A217 (-87.2284, 81.3932) -> (-85.8849, 81.9497) centre (-87.2284, 83.2932) ccw
  line L211 (-83.5565, 84.2781) -> (-85.8849, 81.9497)
  arc A218 (-82.0716, 84.8932) -> (-83.5565, 84.2781) centre (-82.0716, 82.7933) ccw
  line L212 (-82.0716, 84.8932) -> (-64.7284, 84.8932)
  arc A219 (-63.2435, 84.2781) -> (-64.7284, 84.8932) centre (-64.7285, 82.7931) ccw
  line L213 (-63.2435, 84.2781) -> (-59.9151, 80.9497)
  arc A220 (-59.9151, 80.9497) -> (-58.5716, 80.3932) centre (-58.5716, 82.2931) ccw
  line L214 (-58.5716, 80.3932) -> (-45.7284, 80.3932)
  arc A221 (-44.2435, 79.7781) -> (-45.7284, 80.3932) centre (-45.7285, 78.2931) ccw
  line L215 (-43.1151, 78.6497) -> (-44.2435, 79.7781)
  arc A222 (-43.1151, 78.6497) -> (-41.7716, 78.0932) centre (-41.7716, 79.9932) ccw
  line L216 (-41.7716, 78.0932) -> (-8.6, 78.0932)
  arc A223 (-7, 76.4932) -> (-8.6, 78.0932) centre (-8.6, 76.4932) ccw
  line L217 (-7, 1.9932) -> (-7, 76.4932)
  arc A224 (-8.6, 0.3932) -> (-7, 1.9932) centre (-8.6, 1.9932) ccw
  line L218 (-8.6, 0.3932) -> (-25.0716, 0.3932)
  arc A225 (-26.5565, 1.0083) -> (-25.0716, 0.3932) centre (-25.0715, 2.4933) ccw
  line L219 (-26.5565, 1.0083) -> (-27.6849, 2.1367)
  arc A226 (-27.6849, 2.1367) -> (-29.0284, 2.6932) centre (-29.0284, 0.7933) ccw
  line L220 (-44.0716, 2.6932) -> (-29.0284, 2.6932)
  arc A227 (-45.5565, 3.3083) -> (-44.0716, 2.6932) centre (-44.0715, 4.7933) ccw
  line L221 (-45.5565, 3.3083) -> (-46.6849, 4.4367)
  arc A228 (-46.6849, 4.4367) -> (-48.0284, 4.9932) centre (-48.0284, 3.0933) ccw
  line L222 (-48.0284, 4.9932) -> (-62.7328, 4.9932)
  arc A229 (-64.5612, 6.0602) -> (-62.7328, 4.9932) centre (-62.7328, 7.0932) ccw
  line L223 (-64.5612, 6.0602) -> (-72.8388, 20.7116)
  arc A230 (-72.8388, 20.7116) -> (-76.2344, 22.6932) centre (-76.2344, 18.793) ccw
  line L224 (-92.6574, 22.6932) -> (-76.2344, 22.6932)
  arc A231 (-92.6574, 22.6932) -> (-94.708, 21.8438) centre (-92.6573, 19.7931) ccw
  line L225 (-100.9506, 15.6012) -> (-94.708, 21.8438)
  arc A232 (-103.1426, 14.6932) -> (-100.9506, 15.6012) centre (-103.1426, 17.7931) ccw
  line L226 (-138.1, 14.6932) -> (-103.1426, 14.6932)
  arc A233 (-139.7, 16.2932) -> (-138.1, 14.6932) centre (-138.1, 16.2932) ccw
  line L227 (-139.7, 69.4932) -> (-139.7, 16.2932)
  arc A234 (-138.1, 71.0932) -> (-139.7, 69.4932) centre (-138.1, 69.4932) ccw
  line L228 (-138.1, 71.0932) -> (-124.0284, 71.0932)
  arc A235 (-124.0284, 71.0932) -> (-122.6849, 71.6497) centre (-124.0284, 72.9932) ccw
  line L229 (-120.3201, 75.8932) -> (-111.5983, 75.8932)
  line L230 (-101.3201, 83.8932) -> (-88.0983, 83.8932)
  line L231 (-82.3201, 87.3932) -> (-64.4799, 87.3932)
  line L232 (-57.7017, 82.8932) -> (-45.4799, 82.8932)
  line L233 (-40.9017, 80.5932) -> (-8.5, 80.5932)
  line L234 (-4.5, 1.8932) -> (-4.5, 76.5932)
  line L235 (-8.5, -2.1068) -> (-25.3201, -2.1068)
  line L236 (-44.3201, 0.1932) -> (-29.8983, 0.1932)
  line L237 (-48.8983, 2.4932) -> (-63.083, 2.4932)
  line L238 (-91.9946, 20.1932) -> (-77.1681, 20.1932)
  line L239 (-138.2, 12.1932) -> (-102.687, 12.1932)
  line L240 (-142.2, 69.5932) -> (-142.2, 16.1932)
  line L241 (-138.2, 73.5932) -> (-124.8983, 73.5932)
  line L242 (-66.5656, 4.5256) -> (-74.5561, 18.6689)
  line L243 (-99.505, 13.5112) -> (-93.4088, 19.6074)
  arc A236 (-138.2, 73.5932) -> (-142.2, 69.5932) centre (-138.2, 69.5932) ccw
  arc A237 (-142.2, 16.1932) -> (-138.2, 12.1932) centre (-138.2, 16.1932) ccw
  arc A238 (-8.5, -2.1068) -> (-4.5, 1.8932) centre (-8.5, 1.8932) ccw
  arc A239 (-4.5, 76.5932) -> (-8.5, 80.5932) centre (-8.5, 76.5932) ccw
  arc A240 (-111.5983, 75.8932) -> (-110.5376, 76.3325) centre (-111.5983, 77.3932) ccw
  arc A241 (-66.5656, 4.5256) -> (-63.083, 2.4932) centre (-63.083, 6.4932) ccw
  arc A242 (-74.5561, 18.6689) -> (-77.1681, 20.1932) centre (-77.1681, 17.1932) ccw
  arc A243 (-91.9946, 20.1932) -> (-93.4088, 19.6074) centre (-91.9946, 18.1932) ccw
  arc A244 (-102.687, 12.1932) -> (-99.505, 13.5112) centre (-102.687, 16.6932) ccw
  arc A245 (-21.1, 78.0932) -> (-20.3, 77.2932) centre (-20.3, 78.0932) ccw
  arc A246 (-7.8, 39.7932) -> (-7, 38.9932) centre (-7, 39.7932) ccw
  arc A247 (-7.8, 6.3932) -> (-7, 5.5932) centre (-7, 6.3932) ccw
  arc A248 (-7, 13.5932) -> (-7.8, 12.7932) centre (-7, 12.7932) ccw
  arc A249 (-7.8, 76.4932) -> (-8.6, 77.2932) centre (-8.6, 76.4932) ccw
  line L244 (-22.9, 37.8932) -> (-9.9, 37.8932)
  line L245 (-22.9, 34.8932) -> (-9.9, 34.8932)
  line L246 (-24.9, 28.8932) -> (-24.9, 32.8932)
  line L247 (-24.9, 39.8932) -> (-24.9, 73.8932)
  line L248 (-7.9, 73.8932) -> (-7.9, 39.8932)
  line L249 (-7.9, 32.8932) -> (-7.9, 28.8932)
  arc A250 (-24.9, 39.8932) -> (-22.9, 37.8932) centre (-22.9, 39.8932) ccw
  arc A251 (-9.9, 37.8932) -> (-7.9, 39.8932) centre (-9.9, 39.8932) ccw
  arc A252 (-22.9, 34.8932) -> (-24.9, 32.8932) centre (-22.9, 32.8932) ccw
  arc A253 (-7.9, 32.8932) -> (-9.9, 34.8932) centre (-9.9, 32.8932) ccw
  line L250 (-123.8376, 74.0325) -> (-123.1485, 74.7216)
  line L251 (-110.5376, 76.3325) -> (-104.1485, 82.7216)
  line L252 (-87.0376, 84.3325) -> (-85.1485, 86.2216)
  line L253 (-61.6515, 86.2216) -> (-58.7624, 83.3325)
  line L254 (-42.6515, 81.7216) -> (-41.9624, 81.0325)
  line L255 (-28.1485, -0.9352) -> (-28.8376, -0.2461)
  line L256 (-47.8376, 2.0539) -> (-47.1485, 1.3648)
  arc A254 (-47.8376, 2.0539) -> (-48.8983, 2.4932) centre (-48.8983, 0.9932) ccw
  arc A255 (-28.8376, -0.2461) -> (-29.8983, 0.1932) centre (-29.8983, -1.3068) ccw
  arc A256 (-47.1485, 1.3648) -> (-44.3201, 0.1932) centre (-44.3201, 4.1932) ccw
  arc A257 (-28.1485, -0.9352) -> (-25.3201, -2.1068) centre (-25.3201, 1.8932) ccw
  arc A258 (-41.9624, 81.0325) -> (-40.9017, 80.5932) centre (-40.9017, 82.0932) ccw
  arc A259 (-42.6515, 81.7216) -> (-45.4799, 82.8932) centre (-45.4799, 78.8932) ccw
  arc A260 (-82.3201, 87.3932) -> (-85.1485, 86.2216) centre (-82.3201, 83.3932) ccw
  arc A261 (-61.6515, 86.2216) -> (-64.4799, 87.3932) centre (-64.4799, 83.3932) ccw
  arc A262 (-58.7624, 83.3325) -> (-57.7017, 82.8932) centre (-57.7017, 84.3932) ccw
  arc A263 (-88.0983, 83.8932) -> (-87.0376, 84.3325) centre (-88.0983, 85.3932) ccw
  arc A264 (-101.3201, 83.8932) -> (-104.1485, 82.7216) centre (-101.3201, 79.8932) ccw
  arc A265 (-120.3201, 75.8932) -> (-123.1485, 74.7216) centre (-120.3201, 71.8932) ccw
  arc A266 (-124.8983, 73.5932) -> (-123.8376, 74.0325) centre (-124.8983, 75.0932) ccw
  circle A267 centre (-22.6, 22.4932) radius 2.05
  circle A268 centre (-10.1, 22.4932) radius 2.05
  dimension "d1" = 3.3
  dimension "d2" = 3.3
  dimension "d3" = 8
  dimension "d4" = 3.3
  dimension "d5" = 3.3
  dimension "d9" = 2.2
  dimension "d12" = 2.2
  dimension "d318" = 4.1
  dimension "d319" = 4.1
  constraint tangent L19 A5
  constraint tangent L19 A6
  constraint tangent L13 A7
  constraint tangent L17 A8
  constraint tangent L12 A9
  constraint tangent L16 A10
  constraint tangent L8 A11
  constraint tangent L7 A13
  constraint tangent L9 A14
  constraint tangent L18 A15
  constraint tangent L2 A16
  constraint tangent L0 A17
  constraint tangent L10 A18
  constraint tangent L5 A19
  constraint tangent L11 A20
  constraint tangent L6 A21
  constraint tangent L3 A22
  constraint tangent L1 A23
  constraint tangent L4 A24
  constraint tangent L15 A25
  constraint tangent A24 L104
  constraint perpendicular L104 L105
  constraint tangent L104 A26
  constraint tangent L105 A26
  constraint coincident L15.end L105
  constraint perpendicular L15 L105
  constraint coincident L14.end L104
  constraint perpendicular L14 L104
  constraint tangent L32 A27
  constraint tangent L33 A28
  constraint tangent L35 A29
  constraint tangent L34 A30
  constraint tangent L49 A31
  constraint tangent L49 A32
  constraint tangent L51 A33
  constraint tangent L50 A34
  constraint tangent L57 A35
  constraint tangent L57 A36
  constraint tangent L59 A37
  constraint tangent L58 A38
  constraint tangent L76 A39
  constraint tangent L78 A40
  constraint tangent L79 A41
  constraint tangent L77 A42
  constraint tangent L54 A43
  constraint tangent L54 A44
  constraint tangent L52 A45
  constraint tangent L53 A46
  constraint tangent L90 A47
  constraint tangent L90 A48
  constraint tangent L91 A48
  constraint tangent L91 A49
  constraint tangent L89 A50
  constraint tangent L100 A51
  constraint tangent L101 A52
  constraint tangent L103 A53
  constraint tangent L102 A54
  constraint tangent L93 A55
  constraint tangent L93 A56
  constraint tangent L95 A57
  constraint tangent L94 A58
  constraint tangent L21 A59
  constraint tangent L20 A60
  constraint tangent L22 A60
  constraint tangent L22 A61
  constraint tangent L23 A62
  constraint tangent L64 A63
  constraint tangent L66 A63
  constraint tangent L64 A64
  constraint tangent L65 A65
  constraint tangent L67 A66
  constraint tangent L98 A67
  constraint tangent L98 A68
  constraint tangent L96 A69
  constraint tangent L97 A70
  constraint tangent L70 A71
  constraint tangent L70 A72
  constraint tangent L68 A73
  constraint tangent L69 A74
  constraint tangent L80 A75
  constraint tangent L80 A76
  constraint tangent L82 A76
  constraint tangent L82 A77
  constraint tangent L83 A77
  constraint tangent L83 A78
  constraint tangent L81 A78
  constraint tangent L29 A79
  constraint tangent L29 A80
  constraint tangent L28 A81
  constraint tangent L30 A82
  constraint tangent L37 A83
  constraint tangent L37 A84
  constraint tangent L36 A84
  constraint tangent L36 A85
  constraint tangent L38 A85
  constraint tangent L38 A86
  constraint tangent L39 A86
  constraint tangent L61 A87
  constraint tangent L61 A88
  constraint tangent L60 A88
  constraint tangent L60 A89
  constraint tangent L62 A90
  constraint tangent L40 A91
  constraint tangent L42 A92
  constraint tangent L43 A93
  constraint tangent L41 A93
  constraint tangent L41 A94
  constraint tangent L40 A94
  constraint tangent L44 A95
  constraint tangent L46 A95
  constraint tangent L46 A96
  constraint tangent L47 A96
  constraint tangent L47 A97
  constraint tangent L45 A97
  constraint tangent L45 A98
  constraint tangent L44 A98
  constraint tangent L74 A99
  constraint tangent L75 A99
  constraint tangent L74 A100
  constraint tangent L72 A101
  constraint tangent L73 A102
  constraint tangent L26 A103
  constraint tangent L27 A103
  constraint tangent L26 A104
  constraint tangent L24 A105
  constraint tangent L25 A106
  constraint tangent L86 A107
  constraint tangent L87 A107
  constraint tangent L86 A108
  constraint tangent L84 A109
  constraint tangent L85 A110
  constraint tangent A12 L112
  constraint tangent L111 A113
  constraint tangent L112 A113
  constraint concentric A8 A114
  constraint concentric A6 A115
  constraint concentric A23 A116
  constraint concentric A21 A117
  constraint parallel L113 L195
  constraint tangent A118 L195
  constraint tangent L114 A118
  constraint tangent L113 A119
  constraint tangent L113 A120
  constraint tangent L114 A120
  constraint parallel L115 L203
  constraint tangent A123 L203
  constraint tangent L116 A123
  constraint tangent A121 L115
  constraint tangent L115 A122
  constraint tangent A122 L116
  constraint horizontal L117
  constraint perpendicular L117 L118
  constraint parallel L117 L119
  constraint parallel L118 L120
  constraint tangent A127 L120
  constraint tangent L119 A127
  constraint tangent A124 L117
  constraint tangent A124 L120
  constraint tangent L117 A125
  constraint tangent A125 L118
  constraint tangent L118 A126
  constraint tangent A126 L119
  constraint horizontal L121
  constraint perpendicular L121 L122
  constraint parallel L121 L123
  constraint parallel L122 L124
  constraint tangent A131 L124
  constraint tangent L123 A131
  constraint tangent A128 L121
  constraint tangent A128 L124
  constraint tangent L121 A129
  constraint tangent A129 L122
  constraint tangent L122 A130
  constraint tangent A130 L123
  constraint horizontal L125
  constraint perpendicular L125 L198
  constraint parallel L126 L198
  constraint tangent A134 L126
  constraint tangent A132 L125
  constraint tangent A132 L126
  constraint tangent L125 A133
  constraint tangent A133 L198
  constraint horizontal L127
  constraint perpendicular L127 L201
  constraint parallel L128 L201
  constraint tangent A137 L128
  constraint tangent A135 L127
  constraint tangent A135 L128
  constraint tangent L127 A136
  constraint tangent A136 L201
  constraint horizontal L129
  constraint perpendicular L129 L130
  constraint parallel L129 L131
  constraint parallel L130 L132
  constraint tangent A141 L132
  constraint tangent L131 A141
  constraint tangent A138 L129
  constraint tangent A138 L132
  constraint tangent L129 A139
  constraint tangent A139 L130
  constraint tangent L130 A140
  constraint tangent A140 L131
  constraint horizontal L133
  constraint perpendicular L133 L134
  constraint parallel L133 L135
  constraint parallel L134 L136
  constraint tangent A145 L136
  constraint tangent L135 A145
  constraint tangent A142 L133
  constraint tangent A142 L136
  constraint tangent L133 A143
  constraint tangent A143 L134
  constraint tangent L134 A144
  constraint tangent A144 L135
  constraint horizontal L137
  constraint perpendicular L137 L138
  constraint parallel L137 L139
  constraint parallel L138 L140
  constraint tangent A149 L140
  constraint tangent L139 A149
  constraint tangent A146 L137
  constraint tangent A146 L140
  constraint tangent L137 A147
  constraint tangent A147 L138
  constraint tangent L138 A148
  constraint tangent A148 L139
  constraint horizontal L149
  constraint perpendicular L149 L150
  constraint parallel L149 L151
  constraint parallel L150 L152
  constraint tangent A161 L152
  constraint tangent L151 A161
  constraint tangent A158 L149
  constraint tangent A158 L152
  constraint tangent L149 A159
  constraint tangent A159 L150
  constraint tangent L150 A160
  constraint tangent A160 L151
  constraint horizontal L145
  constraint perpendicular L145 L146
  constraint parallel L145 L147
  constraint parallel L146 L148
  constraint tangent A157 L148
  constraint tangent L147 A157
  constraint tangent A154 L145
  constraint tangent A154 L148
  constraint tangent L145 A155
  constraint tangent A155 L146
  constraint tangent L146 A156
  constraint tangent A156 L147
  constraint horizontal L141
  constraint perpendicular L141 L142
  constraint parallel L141 L143
  constraint parallel L142 L144
  constraint tangent A153 L144
  constraint tangent L143 A153
  constraint tangent A150 L141
  constraint tangent A150 L144
  constraint tangent L141 A151
  constraint tangent A151 L142
  constraint tangent L142 A152
  constraint tangent A152 L143
  constraint horizontal L159
  constraint perpendicular L159 L160
  constraint parallel L159 L161
  constraint parallel L160 L162
  constraint tangent A172 L162
  constraint tangent L161 A172
  constraint tangent A169 L159
  constraint tangent A169 L162
  constraint tangent L159 A170
  constraint tangent A170 L160
  constraint tangent L160 A171
  constraint tangent A171 L161
  constraint horizontal L157
  constraint perpendicular L157 L158
  constraint parallel L157 L190
  constraint tangent A166 L157
  constraint tangent L157 A167
  constraint tangent A167 L158
  constraint tangent L158 A168
  constraint tangent A168 L190
  constraint horizontal L153
  constraint perpendicular L153 L154
  constraint parallel L153 L155
  constraint parallel L154 L156
  constraint tangent A165 L156
  constraint tangent L155 A165
  constraint tangent A162 L153
  constraint tangent A162 L156
  constraint tangent L153 A163
  constraint tangent A163 L154
  constraint tangent L154 A164
  constraint tangent A164 L155
  constraint horizontal L163
  constraint perpendicular L163 L164
  constraint parallel L163 L187
  constraint tangent A173 L163
  constraint tangent L163 A174
  constraint tangent A174 L164
  constraint tangent L164 A175
  constraint tangent A175 L187
  constraint horizontal L192
  constraint perpendicular L175 L192
  constraint parallel L176 L192
  constraint parallel L175 L177
  constraint tangent A189 L177
  constraint tangent L176 A189
  constraint tangent A187 L192
  constraint tangent A187 L177
  constraint tangent L175 A188
  constraint tangent A188 L176
  constraint horizontal L171
  constraint perpendicular L171 L172
  constraint parallel L171 L173
  constraint parallel L172 L174
  constraint tangent A186 L174
  constraint tangent L173 A186
  constraint tangent A183 L171
  constraint tangent A183 L174
  constraint tangent L171 A184
  constraint tangent A184 L172
  constraint tangent L172 A185
  constraint tangent A185 L173
  constraint horizontal L185
  constraint parallel L169 L185
  constraint tangent A182 L170
  constraint tangent L169 A182
  constraint tangent A180 L185
  constraint tangent A180 L170
  constraint tangent A181 L169
  constraint horizontal L165
  constraint perpendicular L165 L166
  constraint parallel L165 L167
  constraint parallel L166 L168
  constraint tangent A179 L168
  constraint tangent L167 A179
  constraint tangent A176 L165
  constraint tangent A176 L168
  constraint tangent L165 A177
  constraint tangent A177 L166
  constraint tangent L166 A178
  constraint tangent A178 L167
  constraint horizontal L178
  constraint perpendicular L178 L179
  constraint parallel L178 L180
  constraint parallel L179 L181
  constraint tangent A193 L181
  constraint tangent L180 A193
  constraint tangent A190 L178
  constraint tangent A190 L181
  constraint tangent L178 A191
  constraint tangent A191 L179
  constraint tangent L179 A192
  constraint tangent A192 L180
  constraint horizontal L182
  constraint perpendicular L182 L246
  constraint parallel L182 L183
  constraint parallel L246 L248
  constraint tangent A197 L248
  constraint tangent L183 A197
  constraint tangent A194 L182
  constraint tangent A194 L248
  constraint tangent L182 A195
  constraint tangent A195 L246
  constraint tangent A196 L246
  constraint tangent A196 L183
  constraint parallel L193 L194
  constraint parallel L199 L200
  constraint parallel L205 L206
  constraint tangent L184 A198
  constraint tangent L186 A198
  constraint tangent L185 A199
  constraint tangent L186 A199
  constraint tangent L187 A200
  constraint tangent L189 A200
  constraint tangent L188 A201
  constraint tangent L189 A201
  constraint tangent L190 A202
  constraint tangent L193 A202
  constraint tangent L191 A203
  constraint tangent L193 A203
  constraint tangent L192 A204
  constraint tangent L194 A204
  constraint tangent L175 A205
  constraint tangent L194 A205
  constraint tangent L195 A206
  constraint tangent L199 A206
  constraint tangent L196 A207
  constraint tangent L199 A207
  constraint tangent L197 A208
  constraint tangent L200 A208
  constraint tangent L198 A209
  constraint tangent L200 A209
  constraint tangent L203 A210
  constraint tangent L205 A210
  constraint tangent L204 A211
  constraint tangent L205 A211
  constraint tangent L201 A212
  constraint tangent L206 A212
  constraint tangent L202 A213
  constraint tangent L206 A213
  constraint coincident L233 L107.end
  constraint coincident L234 L106.end
  constraint tangent L240 A236
  constraint tangent L241 A236
  constraint tangent L240 A237
  constraint tangent L239 A237
  constraint tangent L235 A238
  constraint tangent L234 A238
  constraint tangent L233 A239
  constraint tangent L234 A239
  constraint tangent L229 A240
  constraint tangent L237 A241
  constraint tangent L242 A241
  constraint tangent L238 A242
  constraint tangent L242 A242
  constraint tangent L238 A243
  constraint tangent L243 A243
  constraint tangent L239 A244
  constraint tangent L243 A244
  constraint coincident L216 L107.start